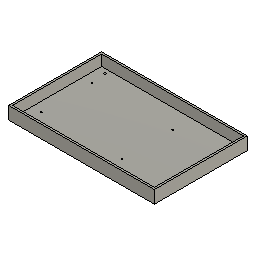
Ensamble Caja con Fuente (Autodesk Fusion 360 archive; units mm, degrees)
design "Caja_Base"
Autodesk Fusion 360 part; units mm, degrees
note: some values were not read from the file. Set by a fixed rule: which face or edge a step refers to.
sketch "Sketch1" plane through (0, 0, 0) normal (0, 0, 1) x (1, 0, 0)
  line L0 (0, 0) -> (229, 0)
  line L1 (229, 0) -> (229, 146)
  line L2 (229, 146) -> (0, 146)
  line L3 (0, 146) -> (0, 0)
  dimension "d1" = 229
  dimension "d2" = 146
  constraint horizontal L0
  constraint vertical L1
  constraint horizontal L2
  constraint vertical L3
  constraint coincident L0.start L3.end
  measures "d1" distance of L0.start L0.end
  measures "d2" distance of L0.end L1.end
extrude "Extrude1" add sketch "Sketch1" along normal blind 20
shell "Shell1" thickness 3 removed faces 1 at (76.3333, 97.3333, 20)
sketch "Sketch2" plane through (0, 0, 0) normal (0, 0, -1) x (1, 0, 0)
  line L0 (0, 0) -> (0, -146)
  line L1 (0, -146) -> (229, -146)
  line L2 (229, -146) -> (229, 0)
  line L3 (229, 0) -> (0, 0)
  circle A0 centre (145.0199, -112.7985) radius 1.25
  line L4 (6.0134, -124.7694) -> (6.0134, -19.8357) construction
  line L5 (205.0199, -127.4985) -> (205.0199, -18.5017) construction
  line L6 (6.0134, -18.5017) -> (6.0134, -127.4985) construction
  line L7 (205.0199, -73) -> (147.0519, -73) construction
  circle A1 centre (18.0134, -112.7985) radius 1.25
  circle A2 centre (18.0134, -33.2015) radius 1.25
  circle A3 centre (145.0199, -33.2015) radius 1.25
  line L8 (6.0134, -127.4985) -> (205.0199, -127.4985) construction
  line L9 (205.0199, -127.4985) -> (9.7448, -127.4985) construction
  line L10 (205.0199, -18.5017) -> (6.0134, -18.5017) construction
  circle A4 centre (15, -136) radius 1.5
  circle A5 centre (214, -136) radius 1.5
  line L11 (210, -73) -> (229, -73) construction
  circle A6 centre (15, -10) radius 1.5
  circle A7 centre (214, -10) radius 1.5
  point P0 (180.3238, -109.2905)
  dimension "d6" = 12
  dimension "d7" = 14.7
  dimension "d8" = 2.5
  dimension "d9" = 108.9968
  dimension "d10" = 54.4985
  dimension "d11" = 2.5
  dimension "d12" = 60
  dimension "d13" = 14.7
  dimension "d15" = 3
  dimension "d16" = 15
  dimension "d17" = 10
  dimension "d18" = 15
  dimension "d19" = 10
  dimension "d20" = 3
  dimension "d21" = 73
  dimension "d24" = 73
  constraint coincident L5.start L8.end
  constraint coincident L7.start L5
  constraint perpendicular L5 L7
  constraint symmetric L7 A1 A2
  constraint symmetric A0 L7 A3
  constraint coincident L2 L11.end
  constraint perpendicular L2 L11
  constraint symmetric A4 L11 A6
  constraint symmetric A5 L11 A7
  measures "d6" distance of A1.centre L4
  measures "d7" distance of A1.centre L9
  measures "d8" diameter of A1
  measures "d9" distance of L8 L10
  measures "d10" distance of L7 L8
  measures "d11" diameter of A0
  measures "d12" distance of A0.centre L5
  measures "d13" distance of A0.centre L8
  measures "d15" diameter of A4
  measures "d16" distance of L0 A4.centre
  measures "d17" distance of L1 A4.centre
  measures "d18" distance of L2 A5.centre
  measures "d19" distance of L1 A5.centre
  measures "d20" diameter of A5
  measures "d21" distance of L1 L11
  measures "d24" distance of L1 L7
extrude "Extrude2" cut sketch "Sketch2" against normal up to surface (3 mm away) contours A0 | A1 | A2 | A3 | A4 | A5 | A6 | A7
equation "d21 = ( 146 / 2 ) * 1 mm"
